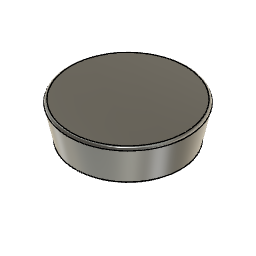
Knob v7 (Autodesk Fusion 360 design; units mm, degrees)
Autodesk Fusion 360 part; units mm, degrees
note: some values were not read from the file. Chosen so that the rebuilt part matches the saved one: which sketch regions a step uses; which face or edge a step refers to.
sketch "Sketch1" plane through (0, 0, 0) normal (0, 0, 1) x (1, 0, 0)
  circle A0 centre (0, 0) radius 5.3
  circle A1 centre (0, 0) radius 2.5
  line L0 (0, 0) -> (0, -1.5)
  line L1 (0, -1.5) -> (-2, -1.5)
  line L2 (0, -1.5) -> (2, -1.5)
  dimension "d1" = 10.6
  dimension "d24" = 5
  dimension "d25" = 1.5
  constraint coincident A0.centre A1.centre
  constraint vertical L0
  constraint coincident A1 L1.end
  constraint perpendicular L0 L1
  constraint coincident A1 L2.end
  constraint perpendicular L0 L2
  measures "d1" diameter of A0
  measures "d24" diameter of A1
  measures "d25" distance of A0.centre L0.end
extrude "Extrude1" add sketch "Sketch1" along normal blind 6 contours A0 | A1 L1 L2 | A1 L1 L2 makes body 1
sketch "Sketch2" plane through (0, 0, 6) normal (0, 0, 1) x (-1, 0, 0)
  circle A0 centre (0, 0) radius 5.3
  circle A1 centre (0, 0) radius 23
  circle A2 centre (0, 0) radius 18
  dimension "d4" = 46
  dimension "d8" = 36
  constraint coincident A0.centre A1.centre
  constraint concentric A1 A2
  measures "d4" diameter of A1
  measures "d8" diameter of A2
extrude "Extrude2" add sketch "Sketch2" along normal blind 16 contours A0 bodies 1
sketch "Sketch3" plane through (0, 0, 22) normal (0, 0, 1) x (-1, 0, 0)
  circle A0 centre (0, 0) radius 5.3
  circle A1 centre (0, 0) radius 26.5
  dimension "d7" = 53
  constraint concentric A0 A1
  measures "d7" diameter of A1
loft "Loft2" add profiles "Sketch2", "Sketch3" section 1 contours A1 | A2 section 2 bodies 1
extrude "Extrude3" cut sketch "Sketch2" along normal blind 12.5 contours A2 bodies 1
fillet "Fillet1" radius 5.5 1 edges at (4.9413, -1.9166, 18.5) on bodies 1
fillet "Fillet2" radius 1 3 edges at (24.7067, -9.5828, 22) (21.4435, 8.3172, 6) (16.7819, 6.5091, 6) on bodies 1
sketch "Sketch4" plane through (0, 0, 6) normal (0, 0, -1) x (1, 0, 0)
  circle A0 centre (0, 0) radius 22.1951
  circle A1 centre (0, 0) radius 19
  circle A2 centre (-108.059, -0.6198) radius 5.35
  dimension "d15" = 10.7
  measures "d15" diameter of A2
extrude "Extrude4" add sketch "Sketch4" along normal blind 7 separate body contours A2 makes body 2
extrude "Extrude5" add 1 faces at (-106.4522, 1.3936, 6) along direction (0, 0, 1) blind 6 on bodies 2 bodies 2
sketch "Sketch5" plane through (0, 0, 12) normal (0, 0, 1) x (-1, 0, 0)
  circle A0 centre (108.059, -0.6198) radius 5.35
  circle A1 centre (108.059, -0.6198) radius 2.75
  line L0 (108.059, -0.6198) -> (108.059, -2.1198)
  line L1 (108.059, -2.1198) -> (110.3638, -2.1198)
  line L2 (108.059, -2.1198) -> (105.7541, -2.1198)
  dimension "d20" = 5.5
  dimension "d21" = 1.5
  constraint concentric A0 A1
  constraint coincident A0.centre A1.centre
  constraint vertical L0
  constraint coincident A1 L1.end
  constraint perpendicular L0 L1
  constraint coincident A1 L2.end
  constraint perpendicular L0 L2
  measures "d20" diameter of A1
  measures "d21" distance of A0.centre L0.end
extrude "Extrude6" cut sketch "Sketch5" against normal blind 11 contours A1 L1 L2 picked at (108.0754, 0.7084) bodies 2
extrude "Extrude7" cut sketch "Sketch1" along normal blind 15 contours A1 L1 L2 picked at (0.0701, 1.1608) bodies 1
sketch "Sketch6" plane through (0, 0, 0) normal (0, 0, 1) x (1, 0, 0)
  circle A0 centre (96.0167, -0.2265) radius 5.3
  dimension "d28" = 10.6
  measures "d28" diameter of A0
extrude "Extrude8" add sketch "Sketch6" along normal blind 6 separate body makes body 3
sketch "Sketch7" plane through (0, 0, 6) normal (0, 0, 1) x (-1, 0, 0)
  circle A0 centre (-96.0167, 0.2265) radius 5.3
  line L0 (-73.017, 0.3402) -> (-84.6153, 20.2016)
  line L1 (-84.6153, 20.2016) -> (-107.6151, 20.0879)
  line L2 (-107.6151, 20.0879) -> (-119.0164, 0.1128)
  line L3 (-119.0164, 0.1128) -> (-107.4181, -19.7487)
  line L4 (-107.4181, -19.7487) -> (-84.4184, -19.635)
  line L5 (-84.4184, -19.635) -> (-73.017, 0.3402)
  point P0 (-96.0167, 0.2265)
  dimension "d31" = 23
  constraint coincident P0 A0.centre
  measures "d31" distance of L0.start P0
extrude "Extrude9" add sketch "Sketch7" along normal blind 22 contours A0 bodies 3
sketch "Sketch8" plane through (0, 0, 28) normal (0, 0, 1) x (-1, 0, 0)
  circle A0 centre (-96.0167, 0.2265) radius 5.3
  line L0 (-69.5167, 0.2265) -> (-82.7667, 23.1761)
  line L1 (-82.7667, 23.1761) -> (-109.2667, 23.1761)
  line L2 (-109.2667, 23.1761) -> (-122.5167, 0.2265)
  line L3 (-122.5167, 0.2265) -> (-109.2667, -22.7232)
  line L4 (-109.2667, -22.7232) -> (-82.7667, -22.7232)
  line L5 (-82.7667, -22.7232) -> (-69.5167, 0.2265)
  point P0 (-96.0167, 0.2265)
  dimension "d34" = 26.5
  constraint coincident P0 A0.centre
  measures "d34" distance of L0.start P0
loft "Loft3" cut profiles "Sketch7", "Sketch8" section 1 contours A0 | L0 L1 L2 L3 L4 L5 section 2 bodies 3
loft "Loft4" add profiles "Sketch7", "Sketch8" section 1 contours A0 | L0 L1 L2 L3 L4 L5 section 2 bodies 3
sketch "Sketch9" plane through (0, 0, 6) normal (0, 0, 1) x (1, 0, 0)
move_body "Move1" bodies 1 to x (1, 0, 0) y (0, 1, 0) z (0, 0, 1) at (-70, 0, 0)
sketch "Sketch10" plane through (0, 0, 0) normal (0, 0, 1) x (1, 0, 0)
  line L0 (0, 0) -> (-4.8705, -3.3615)
  constraint coincident L0.start origin
move_body "Move2" bodies 3 to x (1, 0, 0) y (0, 1, 0) z (0, 0, 1) at (-96.0167, 0.2265, 0)
sketch "Sketch11" plane through (0, 0, 6) normal (0, 0, -1) x (1, 0, 0)
  line L0 (-22.9997, 0.1137) -> (-11.5983, -19.8615)
  line L1 (-11.5983, -19.8615) -> (11.4014, -19.9752)
  line L2 (11.4014, -19.9752) -> (22.9997, -0.1137)
  line L3 (22.9997, -0.1137) -> (11.5983, 19.8615)
  line L4 (11.5983, 19.8615) -> (-11.4014, 19.9752)
  line L5 (-11.4014, 19.9752) -> (-22.9997, 0.1137)
  circle A0 centre (0, 0) radius 5.3
  circle A1 centre (0, 0) radius 15
  dimension "d36" = 30
  constraint coincident A0.centre A1.centre
  measures "d36" diameter of A1
extrude "Extrude10" cut sketch "Sketch11" against normal blind 13 contours A1 bodies 3
sketch "Sketch12" plane through (0, 0, 0) normal (0, 0, -1) x (1, 0, 0)
  circle A0 centre (0, 0) radius 5.3
  circle A1 centre (0, 0) radius 2.5
  line L0 (0, 0) -> (0, 1.5)
  line L1 (0, 1.5) -> (-2, 1.5)
  line L2 (2, 1.5) -> (0, 1.5)
  dimension "d39" = 5
  dimension "d40" = 1.5
  constraint concentric A0 A1
  constraint coincident A0.centre A1.centre
  constraint vertical L0
  constraint coincident A1 L1.end
  constraint perpendicular L0 L1
  constraint coincident A1 L2.start
  constraint perpendicular L0 L2
  measures "d39" diameter of A1
  measures "d40" distance of A0.centre L0.end
extrude "Extrude11" cut sketch "Sketch12" against normal blind 18 contours A1 L1 L2 picked at (0.0701, -1.1608) bodies 3
fillet "Fillet3" radius 1.5 18 edges at (19.875, 11.4748, 28) (0, 22.9497, 28) (-19.875, 11.4748, 28) (-19.875, -11.4748, 28) (0, -22.9497, 28) (19.875, -11.4748, 28) (-24.7499, -0.0569, 17) (-12.4242, 21.4056, 17) (12.3257, 21.4624, 17) (24.7499, 0.0569, 17) (12.4242, -21.4056, 17) (-12.3257, -21.4624, 17) (0.0985, -19.9183, 6) (-17.2006, -10.0444, 6) (17.299, -9.8739, 6) (17.2006, 10.0444, 6) (-0.0985, 19.9183, 6) (-13.9849, -5.4242, 6) on bodies 3
fillet "Fillet4" radius 7.5 1 edges at (-4.9413, 1.9166, 19) on bodies 3
sketch "Sketch13" plane through (0, 0, 0) normal (0, 0, -1) x (1, 0, 0)
  arc A0 (-72, 1.5) -> (-68, 1.5) centre (-70, 0) ccw
  line L0 (-72, 1.5) -> (-68, 1.5)
  circle A1 centre (-70, 0) radius 5.3
  circle A2 centre (-70, 0) radius 3
  line L1 (-70, 0) -> (-70, -3)
  line L2 (-70, -3) -> (-70, 1.8)
  line L3 (-70, 1.8) -> (-67.6, 1.8)
  line L4 (-70, 1.8) -> (-72.4, 1.8)
  dimension "d47" = 4.8
  constraint concentric A0 A2
  constraint coincident A0.centre A1.centre
  constraint coincident A2 L1.end
  constraint vertical L1
  constraint perpendicular L0 L2
  constraint coincident A2 L3.end
  constraint perpendicular L2 L3
  constraint coincident A2 L4.end
  constraint perpendicular L2 L4
  measures "d47" distance of L1.end L2.end
extrude "Extrude12" cut sketch "Sketch13" against normal blind 16 contours A0 L0 A2 L1 L2 L4 | A0 L0 A2 L1 L2 L3 bodies 1
move_face "OffsetFaces1" offset 1.5 2 faces at (-64.7263, 0.5277, 8.3333) (-64.7263, 0.5277, 4) on bodies 1
hidden bodies 2 3
equation "d34 = ( 53 / 2 ) * 1 mm"
